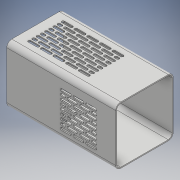
# Autodesk Inventor part: ExtrusionCase
Saved by Autodesk Inventor 2017 (Build 210142000, 142)
## iProperties
Created: 2019-06-19
Part Number: ExtrusionCase
Material: Generic
Document SubType Name: Modeling
Designer: DDeGo
Density: 1 g/cm^3
Appearance: Default
Author: DDeGo
Autodesk Inventor part; units mm, degrees
(part 1 of 2)
ref_plane "YZ Plane" through (0, 0, 0) normal (1, 0, 0) x (0, 1, 0)
ref_plane "XZ Plane" through (0, 0, 0) normal (0, 1, 0) x (-1, 0, 0)
ref_plane "XY Plane" through (0, 0, 0) normal (0, 0, 1) x (1, 0, 0)
sketch "Sketch1" plane through (0, 0, 0) normal (1, 0, 0) x (0, 1, 0)
  line L0 (13, 0) -> (170, 0)
  line L1 (183, -13) -> (183, -170)
  line L2 (170, -183) -> (13, -183)
  line L3 (0, -170) -> (0, -13)
  arc A0 (183, -13) -> (170, 0) centre (170, -13) ccw
  arc A1 (170, -183) -> (183, -170) centre (170, -170) ccw
  arc A2 (0, -170) -> (13, -183) centre (13, -170) ccw
  arc A3 (13, 0) -> (0, -13) centre (13, -13) ccw
  line L4 (186.5, -170) -> (186.5, -13)
  arc A4 (186.5, -13) -> (170, 3.5) centre (170, -13) ccw
  line L5 (170, 3.5) -> (13, 3.5)
  arc A5 (13, 3.5) -> (-3.5, -13) centre (13, -13) ccw
  line L6 (-3.5, -13) -> (-3.5, -170)
  arc A6 (-3.5, -170) -> (13, -186.5) centre (13, -170) ccw
  line L7 (13, -186.5) -> (170, -186.5)
  arc A7 (170, -186.5) -> (186.5, -170) centre (170, -170) ccw
  point P0 (0, 0)
  dimension "d0" = 183
  dimension "d1" = 183
  dimension "d2" = 13
  dimension "d3" = 3.5
  constraints: 16 end point, 16 point on circle, 8 centre point, 8 tangent, 4 parallel, 3 equal radius, 2 perpendicular, 2 point on line, 1 horizontal, 7 other
  measures "d0" distance between parallel lines of L2 L0
  measures "d1" distance between parallel lines of L3 L1
  measures "d2" radius of A0
  measures "d3" distance between parallel lines of L4 L1
extrude "Extrusion1" add sketch "Sketch1" along normal blind 360
sketch "Sketch3" plane through (0, 13, 3.5) normal (0, 0, 1) x (1, 0, 0)
  line L0 (235, 18.5) -> (31, 18.5) construction
  line L1 (31, 18.5) -> (31, 138.5) construction
  line L2 (31, 138.5) -> (235, 138.5) construction
  line L3 (235, 138.5) -> (235, 18.5) construction
  line L4 (0, 157) -> (360, 157) projected
  line L5 (0, 0) -> (360, 0) projected
  line L6 (0, 157) -> (0, 0) projected
  line L7 (230.5556, 134.0556) -> (202.6444, 134.0556) construction
  line L8 (230.5556, 138.5) -> (202.6444, 138.5)
  line L9 (202.6444, 129.6111) -> (230.5556, 129.6111)
  arc A0 (230.5556, 129.6111) -> (230.5556, 138.5) centre (230.5556, 134.0556) ccw
  arc A1 (202.6444, 138.5) -> (202.6444, 129.6111) centre (202.6444, 134.0556) ccw
  line L10 (209.6556, 120.1667) -> (181.7444, 120.1667) construction
  line L11 (209.6556, 124.6111) -> (181.7444, 124.6111)
  line L12 (181.7444, 115.7222) -> (209.6556, 115.7222)
  arc A2 (209.6556, 115.7222) -> (209.6556, 124.6111) centre (209.6556, 120.1667) ccw
  arc A3 (181.7444, 124.6111) -> (181.7444, 115.7222) centre (181.7444, 120.1667) ccw
  arc A4 (202.6444, 110.7222) -> (202.6444, 101.8333) centre (202.6444, 106.2778) ccw
  line L13 (230.5556, 110.7222) -> (202.6444, 110.7222)
  line L14 (202.6444, 101.8333) -> (230.5556, 101.8333)
  arc A5 (230.5556, 101.8333) -> (230.5556, 110.7222) centre (230.5556, 106.2778) ccw
  line L15 (230.5556, 106.2778) -> (202.6444, 106.2778) construction
  arc A6 (202.6444, 82.9444) -> (202.6444, 74.0556) centre (202.6444, 78.5) ccw
  line L16 (230.5556, 82.9444) -> (202.6444, 82.9444)
  line L17 (202.6444, 74.0556) -> (230.5556, 74.0556)
  arc A7 (230.5556, 74.0556) -> (230.5556, 82.9444) centre (230.5556, 78.5) ccw
  line L18 (230.5556, 78.5) -> (202.6444, 78.5) construction
  arc A8 (202.6444, 55.1667) -> (202.6444, 46.2778) centre (202.6444, 50.7222) ccw
  line L19 (230.5556, 55.1667) -> (202.6444, 55.1667)
  line L20 (202.6444, 46.2778) -> (230.5556, 46.2778)
  arc A9 (230.5556, 46.2778) -> (230.5556, 55.1667) centre (230.5556, 50.7222) ccw
  line L21 (230.5556, 50.7222) -> (202.6444, 50.7222) construction
  arc A10 (160.8444, 138.5) -> (160.8444, 129.6111) centre (160.8444, 134.0556) ccw
  line L22 (188.7556, 138.5) -> (160.8444, 138.5)
  line L23 (160.8444, 129.6111) -> (188.7556, 129.6111)
  arc A11 (188.7556, 129.6111) -> (188.7556, 138.5) centre (188.7556, 134.0556) ccw
  line L24 (188.7556, 134.0556) -> (160.8444, 134.0556) construction
  arc A12 (160.8444, 110.7222) -> (160.8444, 101.8333) centre (160.8444, 106.2778) ccw
  line L25 (188.7556, 110.7222) -> (160.8444, 110.7222)
  line L26 (160.8444, 101.8333) -> (188.7556, 101.8333)
  arc A13 (188.7556, 101.8333) -> (188.7556, 110.7222) centre (188.7556, 106.2778) ccw
  line L27 (188.7556, 106.2778) -> (160.8444, 106.2778) construction
  arc A14 (160.8444, 82.9444) -> (160.8444, 74.0556) centre (160.8444, 78.5) ccw
  line L28 (188.7556, 82.9444) -> (160.8444, 82.9444)
  line L29 (160.8444, 74.0556) -> (188.7556, 74.0556)
  arc A15 (188.7556, 74.0556) -> (188.7556, 82.9444) centre (188.7556, 78.5) ccw
  line L30 (188.7556, 78.5) -> (160.8444, 78.5) construction
  arc A16 (160.8444, 55.1667) -> (160.8444, 46.2778) centre (160.8444, 50.7222) ccw
  line L31 (188.7556, 55.1667) -> (160.8444, 55.1667)
  line L32 (160.8444, 46.2778) -> (188.7556, 46.2778)
  arc A17 (188.7556, 46.2778) -> (188.7556, 55.1667) centre (188.7556, 50.7222) ccw
  line L33 (188.7556, 50.7222) -> (160.8444, 50.7222) construction
  arc A18 (119.0444, 138.5) -> (119.0444, 129.6111) centre (119.0444, 134.0556) ccw
  line L34 (146.9556, 138.5) -> (119.0444, 138.5)
  line L35 (119.0444, 129.6111) -> (146.9556, 129.6111)
  arc A19 (146.9556, 129.6111) -> (146.9556, 138.5) centre (146.9556, 134.0556) ccw
  line L36 (146.9556, 134.0556) -> (119.0444, 134.0556) construction
  arc A20 (119.0444, 110.7222) -> (119.0444, 101.8333) centre (119.0444, 106.2778) ccw
  line L37 (146.9556, 110.7222) -> (119.0444, 110.7222)
  line L38 (119.0444, 101.8333) -> (146.9556, 101.8333)
  arc A21 (146.9556, 101.8333) -> (146.9556, 110.7222) centre (146.9556, 106.2778) ccw
  line L39 (146.9556, 106.2778) -> (119.0444, 106.2778) construction
  arc A22 (119.0444, 82.9444) -> (119.0444, 74.0556) centre (119.0444, 78.5) ccw
  line L40 (146.9556, 82.9444) -> (119.0444, 82.9444)
  line L41 (119.0444, 74.0556) -> (146.9556, 74.0556)
  arc A23 (146.9556, 74.0556) -> (146.9556, 82.9444) centre (146.9556, 78.5) ccw
  line L42 (146.9556, 78.5) -> (119.0444, 78.5) construction
  arc A24 (119.0444, 55.1667) -> (119.0444, 46.2778) centre (119.0444, 50.7222) ccw
  line L43 (146.9556, 55.1667) -> (119.0444, 55.1667)
  line L44 (119.0444, 46.2778) -> (146.9556, 46.2778)
  arc A25 (146.9556, 46.2778) -> (146.9556, 55.1667) centre (146.9556, 50.7222) ccw
  line L45 (146.9556, 50.7222) -> (119.0444, 50.7222) construction
  arc A26 (77.2444, 138.5) -> (77.2444, 129.6111) centre (77.2444, 134.0556) ccw
  line L46 (105.1556, 138.5) -> (77.2444, 138.5)
  line L47 (77.2444, 129.6111) -> (105.1556, 129.6111)
  arc A27 (105.1556, 129.6111) -> (105.1556, 138.5) centre (105.1556, 134.0556) ccw
  line L48 (105.1556, 134.0556) -> (77.2444, 134.0556) construction
  arc A28 (77.2444, 110.7222) -> (77.2444, 101.8333) centre (77.2444, 106.2778) ccw
  line L49 (105.1556, 110.7222) -> (77.2444, 110.7222)
  line L50 (77.2444, 101.8333) -> (105.1556, 101.8333)
  arc A29 (105.1556, 101.8333) -> (105.1556, 110.7222) centre (105.1556, 106.2778) ccw
  line L51 (105.1556, 106.2778) -> (77.2444, 106.2778) construction
  arc A30 (77.2444, 82.9444) -> (77.2444, 74.0556) centre (77.2444, 78.5) ccw
  line L52 (105.1556, 82.9444) -> (77.2444, 82.9444)
  line L53 (77.2444, 74.0556) -> (105.1556, 74.0556)
  arc A31 (105.1556, 74.0556) -> (105.1556, 82.9444) centre (105.1556, 78.5) ccw
  line L54 (105.1556, 78.5) -> (77.2444, 78.5) construction
  arc A32 (77.2444, 55.1667) -> (77.2444, 46.2778) centre (77.2444, 50.7222) ccw
  line L55 (105.1556, 55.1667) -> (77.2444, 55.1667)
  line L56 (77.2444, 46.2778) -> (105.1556, 46.2778)
  arc A33 (105.1556, 46.2778) -> (105.1556, 55.1667) centre (105.1556, 50.7222) ccw
  line L57 (105.1556, 50.7222) -> (77.2444, 50.7222) construction
  arc A34 (202.6444, 27.3889) -> (202.6444, 18.5) centre (202.6444, 22.9444) ccw
  line L58 (230.5556, 27.3889) -> (202.6444, 27.3889)
  line L59 (202.6444, 18.5) -> (230.5556, 18.5)
  arc A35 (230.5556, 18.5) -> (230.5556, 27.3889) centre (230.5556, 22.9444) ccw
  line L60 (230.5556, 22.9444) -> (202.6444, 22.9444) construction
  arc A36 (160.8444, 27.3889) -> (160.8444, 18.5) centre (160.8444, 22.9444) ccw
  line L61 (188.7556, 27.3889) -> (160.8444, 27.3889)
  line L62 (160.8444, 18.5) -> (188.7556, 18.5)
  arc A37 (188.7556, 18.5) -> (188.7556, 27.3889) centre (188.7556, 22.9444) ccw
  line L63 (188.7556, 22.9444) -> (160.8444, 22.9444) construction
  arc A38 (119.0444, 27.3889) -> (119.0444, 18.5) centre (119.0444, 22.9444) ccw
  line L64 (146.9556, 27.3889) -> (119.0444, 27.3889)
  line L65 (119.0444, 18.5) -> (146.9556, 18.5)
  arc A39 (146.9556, 18.5) -> (146.9556, 27.3889) centre (146.9556, 22.9444) ccw
  line L66 (146.9556, 22.9444) -> (119.0444, 22.9444) construction
  arc A40 (77.2444, 27.3889) -> (77.2444, 18.5) centre (77.2444, 22.9444) ccw
  line L67 (105.1556, 27.3889) -> (77.2444, 27.3889)
  line L68 (77.2444, 18.5) -> (105.1556, 18.5)
  arc A41 (105.1556, 18.5) -> (105.1556, 27.3889) centre (105.1556, 22.9444) ccw
  line L69 (105.1556, 22.9444) -> (77.2444, 22.9444) construction
  arc A42 (35.4444, 138.5) -> (35.4444, 129.6111) centre (35.4444, 134.0556) ccw
  line L70 (63.3556, 138.5) -> (35.4444, 138.5)
  line L71 (35.4444, 129.6111) -> (63.3556, 129.6111)
  arc A43 (63.3556, 129.6111) -> (63.3556, 138.5) centre (63.3556, 134.0556) ccw
  line L72 (63.3556, 134.0556) -> (35.4444, 134.0556) construction
  arc A44 (35.4444, 110.7222) -> (35.4444, 101.8333) centre (35.4444, 106.2778) ccw
  line L73 (63.3556, 110.7222) -> (35.4444, 110.7222)
  line L74 (35.4444, 101.8333) -> (63.3556, 101.8333)
  arc A45 (63.3556, 101.8333) -> (63.3556, 110.7222) centre (63.3556, 106.2778) ccw
  line L75 (63.3556, 106.2778) -> (35.4444, 106.2778) construction
  arc A46 (35.4444, 82.9444) -> (35.4444, 74.0556) centre (35.4444, 78.5) ccw
  line L76 (63.3556, 82.9444) -> (35.4444, 82.9444)
  line L77 (35.4444, 74.0556) -> (63.3556, 74.0556)
  arc A47 (63.3556, 74.0556) -> (63.3556, 82.9444) centre (63.3556, 78.5) ccw
  line L78 (63.3556, 78.5) -> (35.4444, 78.5) construction
  arc A48 (35.4444, 55.1667) -> (35.4444, 46.2778) centre (35.4444, 50.7222) ccw
  line L79 (63.3556, 55.1667) -> (35.4444, 55.1667)
  line L80 (35.4444, 46.2778) -> (63.3556, 46.2778)
  arc A49 (63.3556, 46.2778) -> (63.3556, 55.1667) centre (63.3556, 50.7222) ccw
  line L81 (63.3556, 50.7222) -> (35.4444, 50.7222) construction
  arc A50 (35.4444, 27.3889) -> (35.4444, 18.5) centre (35.4444, 22.9444) ccw
  line L82 (63.3556, 27.3889) -> (35.4444, 27.3889)
  line L83 (35.4444, 18.5) -> (63.3556, 18.5)
  arc A51 (63.3556, 18.5) -> (63.3556, 27.3889) centre (63.3556, 22.9444) ccw
  line L84 (63.3556, 22.9444) -> (35.4444, 22.9444) construction
  line L85 (216.6, 106.2778) -> (195.7, 120.1667) construction
  line L86 (195.7, 120.1667) -> (174.8, 134.0556) construction
  arc A52 (167.8556, 115.7222) -> (167.8556, 124.6111) centre (167.8556, 120.1667) ccw
  arc A53 (139.9444, 124.6111) -> (139.9444, 115.7222) centre (139.9444, 120.1667) ccw
  line L87 (139.9444, 115.7222) -> (167.8556, 115.7222)
  line L88 (167.8556, 120.1667) -> (139.9444, 120.1667) construction
  line L89 (167.8556, 124.6111) -> (139.9444, 124.6111)
  arc A54 (126.0556, 115.7222) -> (126.0556, 124.6111) centre (126.0556, 120.1667) ccw
  arc A55 (98.1444, 124.6111) -> (98.1444, 115.7222) centre (98.1444, 120.1667) ccw
  line L90 (98.1444, 115.7222) -> (126.0556, 115.7222)
  line L91 (126.0556, 120.1667) -> (98.1444, 120.1667) construction
  line L92 (126.0556, 124.6111) -> (98.1444, 124.6111)
  arc A56 (84.2556, 115.7222) -> (84.2556, 124.6111) centre (84.2556, 120.1667) ccw
  arc A57 (56.3444, 124.6111) -> (56.3444, 115.7222) centre (56.3444, 120.1667) ccw
  line L93 (56.3444, 115.7222) -> (84.2556, 115.7222)
  line L94 (84.2556, 120.1667) -> (56.3444, 120.1667) construction
  line L95 (84.2556, 124.6111) -> (56.3444, 124.6111)
  arc A58 (209.6556, 87.9444) -> (209.6556, 96.8333) centre (209.6556, 92.3889) ccw
  arc A59 (181.7444, 96.8333) -> (181.7444, 87.9444) centre (181.7444, 92.3889) ccw
  line L96 (181.7444, 87.9444) -> (209.6556, 87.9444)
  line L97 (209.6556, 92.3889) -> (181.7444, 92.3889) construction
  line L98 (209.6556, 96.8333) -> (181.7444, 96.8333)
  arc A60 (167.8556, 87.9444) -> (167.8556, 96.8333) centre (167.8556, 92.3889) ccw
  arc A61 (139.9444, 96.8333) -> (139.9444, 87.9444) centre (139.9444, 92.3889) ccw
  line L99 (139.9444, 87.9444) -> (167.8556, 87.9444)
  line L100 (167.8556, 92.3889) -> (139.9444, 92.3889) construction
  line L101 (167.8556, 96.8333) -> (139.9444, 96.8333)
  arc A62 (126.0556, 87.9444) -> (126.0556, 96.8333) centre (126.0556, 92.3889) ccw
  arc A63 (98.1444, 96.8333) -> (98.1444, 87.9444) centre (98.1444, 92.3889) ccw
  line L102 (98.1444, 87.9444) -> (126.0556, 87.9444)
  line L103 (126.0556, 92.3889) -> (98.1444, 92.3889) construction
  line L104 (126.0556, 96.8333) -> (98.1444, 96.8333)
  arc A64 (84.2556, 87.9444) -> (84.2556, 96.8333) centre (84.2556, 92.3889) ccw
  arc A65 (56.3444, 96.8333) -> (56.3444, 87.9444) centre (56.3444, 92.3889) ccw
  line L105 (56.3444, 87.9444) -> (84.2556, 87.9444)
  line L106 (84.2556, 92.3889) -> (56.3444, 92.3889) construction
  line L107 (84.2556, 96.8333) -> (56.3444, 96.8333)
  arc A66 (209.6556, 60.1667) -> (209.6556, 69.0556) centre (209.6556, 64.6111) ccw
  arc A67 (181.7444, 69.0556) -> (181.7444, 60.1667) centre (181.7444, 64.6111) ccw
  line L108 (181.7444, 60.1667) -> (209.6556, 60.1667)
  line L109 (209.6556, 64.6111) -> (181.7444, 64.6111) construction
  line L110 (209.6556, 69.0556) -> (181.7444, 69.0556)
  arc A68 (167.8556, 60.1667) -> (167.8556, 69.0556) centre (167.8556, 64.6111) ccw
  arc A69 (139.9444, 69.0556) -> (139.9444, 60.1667) centre (139.9444, 64.6111) ccw
  line L111 (139.9444, 60.1667) -> (167.8556, 60.1667)
  line L112 (167.8556, 64.6111) -> (139.9444, 64.6111) construction
  line L113 (167.8556, 69.0556) -> (139.9444, 69.0556)
  arc A70 (126.0556, 60.1667) -> (126.0556, 69.0556) centre (126.0556, 64.6111) ccw
  arc A71 (98.1444, 69.0556) -> (98.1444, 60.1667) centre (98.1444, 64.6111) ccw
  line L114 (98.1444, 60.1667) -> (126.0556, 60.1667)
  line L115 (126.0556, 64.6111) -> (98.1444, 64.6111) construction
  line L116 (126.0556, 69.0556) -> (98.1444, 69.0556)
  arc A72 (84.2556, 60.1667) -> (84.2556, 69.0556) centre (84.2556, 64.6111) ccw
  arc A73 (56.3444, 69.0556) -> (56.3444, 60.1667) centre (56.3444, 64.6111) ccw
  line L117 (56.3444, 60.1667) -> (84.2556, 60.1667)
  line L118 (84.2556, 64.6111) -> (56.3444, 64.6111) construction
  line L119 (84.2556, 69.0556) -> (56.3444, 69.0556)
  arc A74 (209.6556, 32.3889) -> (209.6556, 41.2778) centre (209.6556, 36.8333) ccw
  arc A75 (181.7444, 41.2778) -> (181.7444, 32.3889) centre (181.7444, 36.8333) ccw
  line L120 (181.7444, 32.3889) -> (209.6556, 32.3889)
  line L121 (209.6556, 36.8333) -> (181.7444, 36.8333) construction
  line L122 (209.6556, 41.2778) -> (181.7444, 41.2778)
  arc A76 (167.8556, 32.3889) -> (167.8556, 41.2778) centre (167.8556, 36.8333) ccw
  arc A77 (139.9444, 41.2778) -> (139.9444, 32.3889) centre (139.9444, 36.8333) ccw
  line L123 (139.9444, 32.3889) -> (167.8556, 32.3889)
  line L124 (167.8556, 36.8333) -> (139.9444, 36.8333) construction
  line L125 (167.8556, 41.2778) -> (139.9444, 41.2778)
  arc A78 (126.0556, 32.3889) -> (126.0556, 41.2778) centre (126.0556, 36.8333) ccw
  arc A79 (98.1444, 41.2778) -> (98.1444, 32.3889) centre (98.1444, 36.8333) ccw
  line L126 (98.1444, 32.3889) -> (126.0556, 32.3889)
  line L127 (126.0556, 36.8333) -> (98.1444, 36.8333) construction
  line L128 (126.0556, 41.2778) -> (98.1444, 41.2778)
  arc A80 (84.2556, 32.3889) -> (84.2556, 41.2778) centre (84.2556, 36.8333) ccw
  arc A81 (56.3444, 41.2778) -> (56.3444, 32.3889) centre (56.3444, 36.8333) ccw
  line L129 (56.3444, 32.3889) -> (84.2556, 32.3889)
  line L130 (84.2556, 36.8333) -> (56.3444, 36.8333) construction
  line L131 (84.2556, 41.2778) -> (56.3444, 41.2778)
  line L132 (198.2, 134.0556) -> (198.2, 127.2649) construction
  line L133 (193.2, 134.0556) -> (193.2, 126.603) construction
  point P0 (0, -13)
  point P1 (216.6, 134.0556)
  point P2 (235, 110.7222)
  point P3 (235, 82.9444)
  point P4 (216.6, 78.5)
  point P5 (235, 55.1667)
  point P6 (216.6, 50.7222)
  point P7 (193.2, 138.5)
  point P8 (193.2, 110.7222)
  point P9 (174.8, 106.2778)
  point P10 (193.2, 82.9444)
  point P11 (174.8, 78.5)
  point P12 (193.2, 55.1667)
  point P13 (174.8, 50.7222)
  point P14 (151.4, 138.5)
  point P15 (133, 134.0556)
  point P16 (151.4, 110.7222)
  point P17 (133, 106.2778)
  point P18 (151.4, 82.9444)
  point P19 (133, 78.5)
  point P20 (151.4, 55.1667)
  point P21 (133, 50.7222)
  point P22 (109.6, 138.5)
  point P23 (91.2, 134.0556)
  point P24 (109.6, 110.7222)
  point P25 (91.2, 106.2778)
  point P26 (109.6, 82.9444)
  point P27 (91.2, 78.5)
  point P28 (109.6, 55.1667)
  point P29 (91.2, 50.7222)
  point P30 (235, 27.3889)
  point P31 (216.6, 22.9444)
  point P32 (193.2, 27.3889)
  point P33 (174.8, 22.9444)
  point P34 (151.4, 27.3889)
  point P35 (133, 22.9444)
  point P36 (109.6, 27.3889)
  point P37 (91.2, 22.9444)
  point P38 (67.8, 138.5)
  point P39 (49.4, 134.0556)
  point P40 (67.8, 110.7222)
  point P41 (49.4, 106.2778)
  point P42 (67.8, 82.9444)
  point P43 (49.4, 78.5)
  point P44 (67.8, 55.1667)
  point P45 (49.4, 50.7222)
  point P46 (67.8, 27.3889)
  point P47 (49.4, 22.9444)
  point P48 (153.9, 120.1667)
  point P49 (112.1, 120.1667)
  point P50 (70.3, 120.1667)
  point P51 (195.7, 92.3889)
  point P52 (153.9, 92.3889)
  point P53 (112.1, 92.3889)
  point P54 (70.3, 92.3889)
  point P55 (195.7, 64.6111)
  point P56 (153.9, 64.6111)
  point P57 (112.1, 64.6111)
  point P58 (70.3, 64.6111)
  point P59 (195.7, 36.8333)
  point P60 (153.9, 36.8333)
  point P61 (112.1, 36.8333)
  point P62 (70.3, 36.8333)
  dimension "d26" = 18.5
  dimension "d27" = 18.5
  dimension "d28" = 235
  dimension "d29" = 31
  dimension "d37" = 27.7778
  dimension "d40" = 41.8
  dimension "d54" = 41.8
  dimension "d57" = 27.7778
  dimension "d112" = 5
  dimension "d113" = 5
  dimension "d114" = 27.9111
  dimension "d131" = 4.4444
  dimension "d132" = 4.4444
  constraints: 344 end point, 166 point on circle, 82 centre point, 10 tangent, 7 equal length, 5 horizontal, 4 vertical, 2 collinear, 2 midpoint, 1 perpendicular, 492 other
  measures "d26" distance between parallel lines of L2 L4
  measures "d27" distance between parallel lines of L5 L0
  measures "d28" distance between parallel lines of L6 L3
  measures "d29" distance between parallel lines of L6 L1
  measures "d37" distance of L2.end point (235, 110.722)
  measures "d40" distance of L2.end point (193.2, 138.5)
  measures "d54" distance of L10.start L88.start
  measures "d57" distance of L10.start L97.start
  measures "d112" distance between parallel lines of L9 L11
  measures "d113" distance between parallel lines of L133 L132
  measures "d114" distance of L7.start L7.end
  measures "d131" radius of A0
  measures "d132" radius of A2
extrude "Extrusion3" cut sketch "Sketch3" against normal blind 10
sketch "Sketch4" plane through (0, -3.5, -170) normal (0, -1, 0) x (1, 0, 0)
  line L0 (177, 131) -> (297, 131) construction
  line L1 (297, 131) -> (297, 11) construction
  line L2 (297, 11) -> (177, 11) construction
  line L3 (177, 11) -> (177, 131) construction
  line L4 (0, 0) -> (360, 0) projected
  line L5 (0, 157) -> (0, 0) projected
  line L6 (181.4444, 15.4444) -> (209.2222, 15.4444) construction
  line L7 (181.4444, 11) -> (209.2222, 11)
  line L8 (209.2222, 19.8889) -> (181.4444, 19.8889)
  arc A0 (181.4444, 19.8889) -> (181.4444, 11) centre (181.4444, 15.4444) ccw
  arc A1 (209.2222, 11) -> (209.2222, 19.8889) centre (209.2222, 15.4444) ccw
  line L9 (223.1111, 15.4444) -> (250.8889, 15.4444) construction
  line L10 (223.1111, 11) -> (250.8889, 11)
  line L11 (250.8889, 19.8889) -> (223.1111, 19.8889)
  arc A2 (223.1111, 19.8889) -> (223.1111, 11) centre (223.1111, 15.4444) ccw
  arc A3 (250.8889, 11) -> (250.8889, 19.8889) centre (250.8889, 15.4444) ccw
  line L12 (264.7778, 15.4444) -> (292.5556, 15.4444) construction
  line L13 (264.7778, 11) -> (292.5556, 11)
  line L14 (292.5556, 19.8889) -> (264.7778, 19.8889)
  arc A4 (264.7778, 19.8889) -> (264.7778, 11) centre (264.7778, 15.4444) ccw
  arc A5 (292.5556, 11) -> (292.5556, 19.8889) centre (292.5556, 15.4444) ccw
  line L15 (181.4444, 43.2222) -> (209.2222, 43.2222) construction
  line L16 (181.4444, 38.7778) -> (209.2222, 38.7778)
  line L17 (209.2222, 47.6667) -> (181.4444, 47.6667)
  arc A6 (181.4444, 47.6667) -> (181.4444, 38.7778) centre (181.4444, 43.2222) ccw
  arc A7 (209.2222, 38.7778) -> (209.2222, 47.6667) centre (209.2222, 43.2222) ccw
  line L18 (223.1111, 43.2222) -> (250.8889, 43.2222) construction
  line L19 (223.1111, 38.7778) -> (250.8889, 38.7778)
  line L20 (250.8889, 47.6667) -> (223.1111, 47.6667)
  arc A8 (223.1111, 47.6667) -> (223.1111, 38.7778) centre (223.1111, 43.2222) ccw
  arc A9 (250.8889, 38.7778) -> (250.8889, 47.6667) centre (250.8889, 43.2222) ccw
  line L21 (264.7778, 43.2222) -> (292.5556, 43.2222) construction
  line L22 (264.7778, 38.7778) -> (292.5556, 38.7778)
  line L23 (292.5556, 47.6667) -> (264.7778, 47.6667)
  arc A10 (264.7778, 47.6667) -> (264.7778, 38.7778) centre (264.7778, 43.2222) ccw
  arc A11 (292.5556, 38.7778) -> (292.5556, 47.6667) centre (292.5556, 43.2222) ccw
  line L24 (181.4444, 71) -> (209.2222, 71) construction
  line L25 (181.4444, 66.5556) -> (209.2222, 66.5556)
  line L26 (209.2222, 75.4444) -> (181.4444, 75.4444)
  arc A12 (181.4444, 75.4444) -> (181.4444, 66.5556) centre (181.4444, 71) ccw
  arc A13 (209.2222, 66.5556) -> (209.2222, 75.4444) centre (209.2222, 71) ccw
  line L27 (223.1111, 71) -> (250.8889, 71) construction
  line L28 (223.1111, 66.5556) -> (250.8889, 66.5556)
  line L29 (250.8889, 75.4444) -> (223.1111, 75.4444)
  arc A14 (223.1111, 75.4444) -> (223.1111, 66.5556) centre (223.1111, 71) ccw
  arc A15 (250.8889, 66.5556) -> (250.8889, 75.4444) centre (250.8889, 71) ccw
  line L30 (264.7778, 71) -> (292.5556, 71) construction
  line L31 (264.7778, 66.5556) -> (292.5556, 66.5556)
  line L32 (292.5556, 75.4444) -> (264.7778, 75.4444)
  arc A16 (264.7778, 75.4444) -> (264.7778, 66.5556) centre (264.7778, 71) ccw
  arc A17 (292.5556, 66.5556) -> (292.5556, 75.4444) centre (292.5556, 71) ccw
  line L33 (181.4444, 98.7778) -> (209.2222, 98.7778) construction
  line L34 (181.4444, 94.3333) -> (209.2222, 94.3333)
  line L35 (209.2222, 103.2222) -> (181.4444, 103.2222)
  arc A18 (181.4444, 103.2222) -> (181.4444, 94.3333) centre (181.4444, 98.7778) ccw
  arc A19 (209.2222, 94.3333) -> (209.2222, 103.2222) centre (209.2222, 98.7778) ccw
  line L36 (223.1111, 98.7778) -> (250.8889, 98.7778) construction
  line L37 (223.1111, 94.3333) -> (250.8889, 94.3333)
  line L38 (250.8889, 103.2222) -> (223.1111, 103.2222)
  arc A20 (223.1111, 103.2222) -> (223.1111, 94.3333) centre (223.1111, 98.7778) ccw
  arc A21 (250.8889, 94.3333) -> (250.8889, 103.2222) centre (250.8889, 98.7778) ccw
  line L39 (264.7778, 98.7778) -> (292.5556, 98.7778) construction
  line L40 (264.7778, 94.3333) -> (292.5556, 94.3333)
  line L41 (292.5556, 103.2222) -> (264.7778, 103.2222)
  arc A22 (264.7778, 103.2222) -> (264.7778, 94.3333) centre (264.7778, 98.7778) ccw
  arc A23 (292.5556, 94.3333) -> (292.5556, 103.2222) centre (292.5556, 98.7778) ccw
  line L42 (181.4444, 126.5556) -> (209.2222, 126.5556) construction
  line L43 (181.4444, 122.1111) -> (209.2222, 122.1111)
  line L44 (209.2222, 131) -> (181.4444, 131)
  arc A24 (181.4444, 131) -> (181.4444, 122.1111) centre (181.4444, 126.5556) ccw
  arc A25 (209.2222, 122.1111) -> (209.2222, 131) centre (209.2222, 126.5556) ccw
  line L45 (223.1111, 126.5556) -> (250.8889, 126.5556) construction
  line L46 (223.1111, 122.1111) -> (250.8889, 122.1111)
  line L47 (250.8889, 131) -> (223.1111, 131)
  arc A26 (223.1111, 131) -> (223.1111, 122.1111) centre (223.1111, 126.5556) ccw
  arc A27 (250.8889, 122.1111) -> (250.8889, 131) centre (250.8889, 126.5556) ccw
  line L48 (264.7778, 126.5556) -> (292.5556, 126.5556) construction
  line L49 (264.7778, 122.1111) -> (292.5556, 122.1111)
  line L50 (292.5556, 131) -> (264.7778, 131)
  arc A28 (264.7778, 131) -> (264.7778, 122.1111) centre (264.7778, 126.5556) ccw
  arc A29 (292.5556, 122.1111) -> (292.5556, 131) centre (292.5556, 126.5556) ccw
  line L51 (203.6667, 29.3333) -> (228.6667, 29.3333) construction
  line L52 (203.6667, 24.8889) -> (228.6667, 24.8889)
  line L53 (228.6667, 33.7778) -> (203.6667, 33.7778)
  arc A30 (203.6667, 33.7778) -> (203.6667, 24.8889) centre (203.6667, 29.3333) ccw
  arc A31 (228.6667, 24.8889) -> (228.6667, 33.7778) centre (228.6667, 29.3333) ccw
  line L54 (195.3333, 43.2222) -> (216.1667, 29.3333) construction
  line L55 (216.1667, 29.3333) -> (237, 15.4444) construction
  arc A32 (270.3333, 24.8889) -> (270.3333, 33.7778) centre (270.3333, 29.3333) ccw
  line L56 (245.3333, 24.8889) -> (270.3333, 24.8889)
  line L57 (245.3333, 29.3333) -> (270.3333, 29.3333) construction
  line L58 (270.3333, 33.7778) -> (245.3333, 33.7778)
  arc A33 (245.3333, 33.7778) -> (245.3333, 24.8889) centre (245.3333, 29.3333) ccw
  arc A34 (228.6667, 52.6667) -> (228.6667, 61.5556) centre (228.6667, 57.1111) ccw
  line L59 (203.6667, 52.6667) -> (228.6667, 52.6667)
  line L60 (203.6667, 57.1111) -> (228.6667, 57.1111) construction
  line L61 (228.6667, 61.5556) -> (203.6667, 61.5556)
  arc A35 (203.6667, 61.5556) -> (203.6667, 52.6667) centre (203.6667, 57.1111) ccw
  arc A36 (270.3333, 52.6667) -> (270.3333, 61.5556) centre (270.3333, 57.1111) ccw
  line L62 (245.3333, 52.6667) -> (270.3333, 52.6667)
  line L63 (245.3333, 57.1111) -> (270.3333, 57.1111) construction
  line L64 (270.3333, 61.5556) -> (245.3333, 61.5556)
  arc A37 (245.3333, 61.5556) -> (245.3333, 52.6667) centre (245.3333, 57.1111) ccw
  arc A38 (228.6667, 80.4444) -> (228.6667, 89.3333) centre (228.6667, 84.8889) ccw
  line L65 (203.6667, 80.4444) -> (228.6667, 80.4444)
  line L66 (203.6667, 84.8889) -> (228.6667, 84.8889) construction
  line L67 (228.6667, 89.3333) -> (203.6667, 89.3333)
  arc A39 (203.6667, 89.3333) -> (203.6667, 80.4444) centre (203.6667, 84.8889) ccw
  arc A40 (270.3333, 80.4444) -> (270.3333, 89.3333) centre (270.3333, 84.8889) ccw
  line L68 (245.3333, 80.4444) -> (270.3333, 80.4444)
  line L69 (245.3333, 84.8889) -> (270.3333, 84.8889) construction
  line L70 (270.3333, 89.3333) -> (245.3333, 89.3333)
  arc A41 (245.3333, 89.3333) -> (245.3333, 80.4444) centre (245.3333, 84.8889) ccw
  arc A42 (228.6667, 108.2222) -> (228.6667, 117.1111) centre (228.6667, 112.6667) ccw
  line L71 (203.6667, 108.2222) -> (228.6667, 108.2222)
  line L72 (203.6667, 112.6667) -> (228.6667, 112.6667) construction
  line L73 (228.6667, 117.1111) -> (203.6667, 117.1111)
  arc A43 (203.6667, 117.1111) -> (203.6667, 108.2222) centre (203.6667, 112.6667) ccw
  arc A44 (270.3333, 108.2222) -> (270.3333, 117.1111) centre (270.3333, 112.6667) ccw
  line L74 (245.3333, 108.2222) -> (270.3333, 108.2222)
  line L75 (245.3333, 112.6667) -> (270.3333, 112.6667) construction
  line L76 (270.3333, 117.1111) -> (245.3333, 117.1111)
  arc A45 (245.3333, 117.1111) -> (245.3333, 108.2222) centre (245.3333, 112.6667) ccw
  line L77 (213.6667, 15.4444) -> (213.6667, 19.5521) construction
  line L78 (218.6667, 15.4444) -> (218.6667, 18.8098) construction
  point P0 (0, 170)
  point P1 (195.3333, 15.4444)
  point P2 (218.6667, 11)
  point P3 (260.3333, 11)
  point P4 (278.6667, 15.4444)
  point P5 (177, 38.7778)
  point P6 (218.6667, 38.7778)
  point P7 (237, 43.2222)
  point P8 (260.3333, 38.7778)
  point P9 (278.6667, 43.2222)
  point P10 (177, 66.5556)
  point P11 (195.3333, 71)
  point P12 (218.6667, 66.5556)
  point P13 (237, 71)
  point P14 (260.3333, 66.5556)
  point P15 (278.6667, 71)
  point P16 (177, 94.3333)
  point P17 (195.3333, 98.7778)
  point P18 (218.6667, 94.3333)
  point P19 (237, 98.7778)
  point P20 (260.3333, 94.3333)
  point P21 (278.6667, 98.7778)
  point P22 (177, 122.1111)
  point P23 (195.3333, 126.5556)
  point P24 (218.6667, 122.1111)
  point P25 (237, 126.5556)
  point P26 (260.3333, 122.1111)
  point P27 (278.6667, 126.5556)
  point P28 (257.8333, 29.3333)
  point P29 (216.1667, 57.1111)
  point P30 (257.8333, 57.1111)
  point P31 (216.1667, 84.8889)
  point P32 (257.8333, 84.8889)
  point P33 (216.1667, 112.6667)
  point P34 (257.8333, 112.6667)
  dimension "d60" = 120
  dimension "d61" = 120
  dimension "d62" = 11
  dimension "d63" = 177
  dimension "d68" = 41.6667
  dimension "d71" = 27.7778
  dimension "d74" = 25
  dimension "d78" = 41.6667
  dimension "d81" = 27.7778
  dimension "d110" = 5
  dimension "d111" = 27.7778
  dimension "d128" = 5
  dimension "d129" = 4.4444
  dimension "d130" = 4.4444
  constraints: 200 end point, 94 point on circle, 46 centre point, 11 tangent, 5 equal length, 5 horizontal, 4 vertical, 3 collinear, 2 midpoint, 1 perpendicular, 266 other
  measures "d60" distance between parallel lines of L3 L1
  measures "d61" distance between parallel lines of L0 L2
  measures "d62" distance between parallel lines of L4 L2
  measures "d63" distance between parallel lines of L5 L3
  measures "d68" distance of L2.end point (218.667, 11)
  measures "d71" distance of L2.end point (177, 38.778)
  measures "d74" distance of L51.start L51.end
  measures "d78" distance of L52.end L56.end
  measures "d81" distance of L52.end L59.end
  measures "d110" distance between parallel lines of L78 L77
  measures "d111" distance of L6.start L6.end
  measures "d128" distance between parallel lines of L8 L52
  measures "d129" radius of A0
  measures "d130" radius of A30
extrude "Extrusion4" cut sketch "Sketch4" against normal blind 10
sketch "Sketch5" plane through (0, 13, -186.5) normal (0, 0, -1) x (-1, 0, 0)
  line L0 (-12, 10) -> (-142, 10) construction
  line L1 (-142, 10) -> (-142, 147) construction
  line L2 (-142, 147) -> (-12, 147) construction
  line L3 (-12, 147) -> (-12, 10) construction
  line L4 (0, 0) -> (-360, 0) projected
  line L5 (0, 157) -> (-360, 157) projected
  line L6 (0, 0) -> (0, 157) projected
  line L7 (-138.0455, 13.9545) -> (-105.9545, 13.9545) construction
  line L8 (-138.0455, 10) -> (-105.9545, 10)
  line L9 (-105.9545, 17.9091) -> (-138.0455, 17.9091)
  arc A0 (-138.0455, 17.9091) -> (-138.0455, 10) centre (-138.0455, 13.9545) ccw
  arc A1 (-105.9545, 10) -> (-105.9545, 17.9091) centre (-105.9545, 13.9545) ccw
  line L10 (-115.5455, 26.8636) -> (-83.4545, 26.8636) construction
  line L11 (-77.2444, 27.3889) -> (-105.1556, 27.3889) construction
  line L12 (-115.5455, 22.9091) -> (-83.4545, 22.9091)
  line L13 (-83.4545, 30.8182) -> (-115.5455, 30.8182)
  arc A2 (-115.5455, 30.8182) -> (-115.5455, 22.9091) centre (-115.5455, 26.8636) ccw
  arc A3 (-83.4545, 22.9091) -> (-83.4545, 30.8182) centre (-83.4545, 26.8636) ccw
  arc A4 (-60.9545, 10) -> (-60.9545, 17.9091) centre (-60.9545, 13.9545) ccw
  line L14 (-60.9545, 17.9091) -> (-93.0455, 17.9091)
  line L15 (-93.0455, 13.9545) -> (-60.9545, 13.9545) construction
  line L16 (-93.0455, 10) -> (-60.9545, 10)
  arc A5 (-93.0455, 17.9091) -> (-93.0455, 10) centre (-93.0455, 13.9545) ccw
  arc A6 (-105.9545, 35.8182) -> (-105.9545, 43.7273) centre (-105.9545, 39.7727) ccw
  line L17 (-105.9545, 43.7273) -> (-138.0455, 43.7273)
  line L18 (-138.0455, 39.7727) -> (-105.9545, 39.7727) construction
  line L19 (-138.0455, 35.8182) -> (-105.9545, 35.8182)
  arc A7 (-138.0455, 43.7273) -> (-138.0455, 35.8182) centre (-138.0455, 39.7727) ccw
  arc A8 (-60.9545, 35.8182) -> (-60.9545, 43.7273) centre (-60.9545, 39.7727) ccw
  line L20 (-60.9545, 43.7273) -> (-93.0455, 43.7273)
  line L21 (-93.0455, 39.7727) -> (-60.9545, 39.7727) construction
  line L22 (-93.0455, 35.8182) -> (-60.9545, 35.8182)
  arc A9 (-93.0455, 43.7273) -> (-93.0455, 35.8182) centre (-93.0455, 39.7727) ccw
  arc A10 (-15.9545, 10) -> (-15.9545, 17.9091) centre (-15.9545, 13.9545) ccw
  line L23 (-15.9545, 17.9091) -> (-48.0455, 17.9091)
  line L24 (-48.0455, 13.9545) -> (-15.9545, 13.9545) construction
  line L25 (-48.0455, 10) -> (-15.9545, 10)
  arc A11 (-48.0455, 17.9091) -> (-48.0455, 10) centre (-48.0455, 13.9545) ccw
  arc A12 (-15.9545, 35.8182) -> (-15.9545, 43.7273) centre (-15.9545, 39.7727) ccw
  line L26 (-15.9545, 43.7273) -> (-48.0455, 43.7273)
  line L27 (-48.0455, 39.7727) -> (-15.9545, 39.7727) construction
  line L28 (-48.0455, 35.8182) -> (-15.9545, 35.8182)
  arc A13 (-48.0455, 43.7273) -> (-48.0455, 35.8182) centre (-48.0455, 39.7727) ccw
  arc A14 (-105.9545, 61.6364) -> (-105.9545, 69.5455) centre (-105.9545, 65.5909) ccw
  line L29 (-105.9545, 69.5455) -> (-138.0455, 69.5455)
  line L30 (-138.0455, 65.5909) -> (-105.9545, 65.5909) construction
  line L31 (-138.0455, 61.6364) -> (-105.9545, 61.6364)
  arc A15 (-138.0455, 69.5455) -> (-138.0455, 61.6364) centre (-138.0455, 65.5909) ccw
  arc A16 (-60.9545, 61.6364) -> (-60.9545, 69.5455) centre (-60.9545, 65.5909) ccw
  line L32 (-60.9545, 69.5455) -> (-93.0455, 69.5455)
  line L33 (-93.0455, 65.5909) -> (-60.9545, 65.5909) construction
  line L34 (-93.0455, 61.6364) -> (-60.9545, 61.6364)
  arc A17 (-93.0455, 69.5455) -> (-93.0455, 61.6364) centre (-93.0455, 65.5909) ccw
  arc A18 (-15.9545, 61.6364) -> (-15.9545, 69.5455) centre (-15.9545, 65.5909) ccw
  line L35 (-15.9545, 69.5455) -> (-48.0455, 69.5455)
  line L36 (-48.0455, 65.5909) -> (-15.9545, 65.5909) construction
  line L37 (-48.0455, 61.6364) -> (-15.9545, 61.6364)
  arc A19 (-48.0455, 69.5455) -> (-48.0455, 61.6364) centre (-48.0455, 65.5909) ccw
  arc A20 (-105.9545, 87.4545) -> (-105.9545, 95.3636) centre (-105.9545, 91.4091) ccw
  line L38 (-105.9545, 95.3636) -> (-138.0455, 95.3636)
  line L39 (-138.0455, 91.4091) -> (-105.9545, 91.4091) construction
  line L40 (-138.0455, 87.4545) -> (-105.9545, 87.4545)
  arc A21 (-138.0455, 95.3636) -> (-138.0455, 87.4545) centre (-138.0455, 91.4091) ccw
  arc A22 (-60.9545, 87.4545) -> (-60.9545, 95.3636) centre (-60.9545, 91.4091) ccw
  line L41 (-60.9545, 95.3636) -> (-93.0455, 95.3636)
  line L42 (-93.0455, 91.4091) -> (-60.9545, 91.4091) construction
  line L43 (-93.0455, 87.4545) -> (-60.9545, 87.4545)
  arc A23 (-93.0455, 95.3636) -> (-93.0455, 87.4545) centre (-93.0455, 91.4091) ccw
  arc A24 (-15.9545, 87.4545) -> (-15.9545, 95.3636) centre (-15.9545, 91.4091) ccw
  line L44 (-15.9545, 95.3636) -> (-48.0455, 95.3636)
  line L45 (-48.0455, 91.4091) -> (-15.9545, 91.4091) construction
  line L46 (-48.0455, 87.4545) -> (-15.9545, 87.4545)
  arc A25 (-48.0455, 95.3636) -> (-48.0455, 87.4545) centre (-48.0455, 91.4091) ccw
  arc A26 (-105.9545, 113.2727) -> (-105.9545, 121.1818) centre (-105.9545, 117.2273) ccw
  line L47 (-105.9545, 121.1818) -> (-138.0455, 121.1818)
  line L48 (-138.0455, 117.2273) -> (-105.9545, 117.2273) construction
  line L49 (-138.0455, 113.2727) -> (-105.9545, 113.2727)
  arc A27 (-138.0455, 121.1818) -> (-138.0455, 113.2727) centre (-138.0455, 117.2273) ccw
  arc A28 (-60.9545, 113.2727) -> (-60.9545, 121.1818) centre (-60.9545, 117.2273) ccw
  line L50 (-60.9545, 121.1818) -> (-93.0455, 121.1818)
  line L51 (-93.0455, 117.2273) -> (-60.9545, 117.2273) construction
  line L52 (-93.0455, 113.2727) -> (-60.9545, 113.2727)
  arc A29 (-93.0455, 121.1818) -> (-93.0455, 113.2727) centre (-93.0455, 117.2273) ccw
  arc A30 (-15.9545, 113.2727) -> (-15.9545, 121.1818) centre (-15.9545, 117.2273) ccw
  line L53 (-15.9545, 121.1818) -> (-48.0455, 121.1818)
  line L54 (-48.0455, 117.2273) -> (-15.9545, 117.2273) construction
  line L55 (-48.0455, 113.2727) -> (-15.9545, 113.2727)
  arc A31 (-48.0455, 121.1818) -> (-48.0455, 113.2727) centre (-48.0455, 117.2273) ccw
  arc A32 (-105.9545, 139.0909) -> (-105.9545, 147) centre (-105.9545, 143.0455) ccw
  line L56 (-105.9545, 147) -> (-138.0455, 147)
  line L57 (-138.0455, 143.0455) -> (-105.9545, 143.0455) construction
  line L58 (-138.0455, 139.0909) -> (-105.9545, 139.0909)
  arc A33 (-138.0455, 147) -> (-138.0455, 139.0909) centre (-138.0455, 143.0455) ccw
  arc A34 (-60.9545, 139.0909) -> (-60.9545, 147) centre (-60.9545, 143.0455) ccw
  line L59 (-60.9545, 147) -> (-93.0455, 147)
  line L60 (-93.0455, 143.0455) -> (-60.9545, 143.0455) construction
  line L61 (-93.0455, 139.0909) -> (-60.9545, 139.0909)
  arc A35 (-93.0455, 147) -> (-93.0455, 139.0909) centre (-93.0455, 143.0455) ccw
  arc A36 (-15.9545, 139.0909) -> (-15.9545, 147) centre (-15.9545, 143.0455) ccw
  line L62 (-15.9545, 147) -> (-48.0455, 147)
  line L63 (-48.0455, 143.0455) -> (-15.9545, 143.0455) construction
  line L64 (-48.0455, 139.0909) -> (-15.9545, 139.0909)
  arc A37 (-48.0455, 147) -> (-48.0455, 139.0909) centre (-48.0455, 143.0455) ccw
  line L65 (-122, 39.7727) -> (-99.5, 26.8636) construction
  line L66 (-99.5, 26.8636) -> (-77, 13.9545) construction
  line L67 (-70.5455, 26.8636) -> (-38.4545, 26.8636) construction
  line L68 (-70.5455, 22.9091) -> (-38.4545, 22.9091)
  line L69 (-38.4545, 30.8182) -> (-70.5455, 30.8182)
  arc A38 (-70.5455, 30.8182) -> (-70.5455, 22.9091) centre (-70.5455, 26.8636) ccw
  arc A39 (-38.4545, 22.9091) -> (-38.4545, 30.8182) centre (-38.4545, 26.8636) ccw
  line L70 (-115.5455, 52.6818) -> (-83.4545, 52.6818) construction
  line L71 (-115.5455, 48.7273) -> (-83.4545, 48.7273)
  line L72 (-83.4545, 56.6364) -> (-115.5455, 56.6364)
  arc A40 (-115.5455, 56.6364) -> (-115.5455, 48.7273) centre (-115.5455, 52.6818) ccw
  arc A41 (-83.4545, 48.7273) -> (-83.4545, 56.6364) centre (-83.4545, 52.6818) ccw
  line L73 (-70.5455, 52.6818) -> (-38.4545, 52.6818) construction
  line L74 (-70.5455, 48.7273) -> (-38.4545, 48.7273)
  line L75 (-38.4545, 56.6364) -> (-70.5455, 56.6364)
  arc A42 (-70.5455, 56.6364) -> (-70.5455, 48.7273) centre (-70.5455, 52.6818) ccw
  arc A43 (-38.4545, 48.7273) -> (-38.4545, 56.6364) centre (-38.4545, 52.6818) ccw
  line L76 (-115.5455, 78.5) -> (-83.4545, 78.5) construction
  line L77 (-115.5455, 74.5455) -> (-83.4545, 74.5455)
  line L78 (-83.4545, 82.4545) -> (-115.5455, 82.4545)
  arc A44 (-115.5455, 82.4545) -> (-115.5455, 74.5455) centre (-115.5455, 78.5) ccw
  arc A45 (-83.4545, 74.5455) -> (-83.4545, 82.4545) centre (-83.4545, 78.5) ccw
  line L79 (-70.5455, 78.5) -> (-38.4545, 78.5) construction
  line L80 (-70.5455, 74.5455) -> (-38.4545, 74.5455)
  line L81 (-38.4545, 82.4545) -> (-70.5455, 82.4545)
  arc A46 (-70.5455, 82.4545) -> (-70.5455, 74.5455) centre (-70.5455, 78.5) ccw
  arc A47 (-38.4545, 74.5455) -> (-38.4545, 82.4545) centre (-38.4545, 78.5) ccw
  line L82 (-115.5455, 104.3182) -> (-83.4545, 104.3182) construction
  line L83 (-115.5455, 100.3636) -> (-83.4545, 100.3636)
  line L84 (-83.4545, 108.2727) -> (-115.5455, 108.2727)
  arc A48 (-115.5455, 108.2727) -> (-115.5455, 100.3636) centre (-115.5455, 104.3182) ccw
  arc A49 (-83.4545, 100.3636) -> (-83.4545, 108.2727) centre (-83.4545, 104.3182) ccw
  line L85 (-70.5455, 104.3182) -> (-38.4545, 104.3182) construction
  line L86 (-70.5455, 100.3636) -> (-38.4545, 100.3636)
  line L87 (-38.4545, 108.2727) -> (-70.5455, 108.2727)
  arc A50 (-70.5455, 108.2727) -> (-70.5455, 100.3636) centre (-70.5455, 104.3182) ccw
  arc A51 (-38.4545, 100.3636) -> (-38.4545, 108.2727) centre (-38.4545, 104.3182) ccw
  line L88 (-115.5455, 130.1364) -> (-83.4545, 130.1364) construction
  line L89 (-115.5455, 126.1818) -> (-83.4545, 126.1818)
  line L90 (-83.4545, 134.0909) -> (-115.5455, 134.0909)
  arc A52 (-115.5455, 134.0909) -> (-115.5455, 126.1818) centre (-115.5455, 130.1364) ccw
  arc A53 (-83.4545, 126.1818) -> (-83.4545, 134.0909) centre (-83.4545, 130.1364) ccw
  line L91 (-70.5455, 130.1364) -> (-38.4545, 130.1364) construction
  line L92 (-70.5455, 126.1818) -> (-38.4545, 126.1818)
  line L93 (-38.4545, 134.0909) -> (-70.5455, 134.0909)
  arc A54 (-70.5455, 134.0909) -> (-70.5455, 126.1818) centre (-70.5455, 130.1364) ccw
  arc A55 (-38.4545, 126.1818) -> (-38.4545, 134.0909) centre (-38.4545, 130.1364) ccw
  line L94 (-102, 13.9545) -> (-102, 22.25) construction
  line L95 (-97, 13.9545) -> (-97, 20.9047) construction
  point P0 (0, -13)
  point P1 (-122, 13.9545)
  point P2 (-97, 10)
  point P3 (-142, 35.8182)
  point P4 (-77, 39.7727)
  point P5 (-97, 35.8182)
  point P6 (-32, 13.9545)
  point P7 (-52, 10)
  point P8 (-32, 39.7727)
  point P9 (-52, 35.8182)
  point P10 (-122, 65.5909)
  point P11 (-142, 61.6364)
  point P12 (-77, 65.5909)
  point P13 (-97, 61.6364)
  point P14 (-32, 65.5909)
  point P15 (-52, 61.6364)
  point P16 (-122, 91.4091)
  point P17 (-142, 87.4545)
  point P18 (-77, 91.4091)
  point P19 (-97, 87.4545)
  point P20 (-32, 91.4091)
  point P21 (-52, 87.4545)
  point P22 (-122, 117.2273)
  point P23 (-142, 113.2727)
  point P24 (-77, 117.2273)
  point P25 (-97, 113.2727)
  point P26 (-32, 117.2273)
  point P27 (-52, 113.2727)
  point P28 (-122, 143.0455)
  point P29 (-142, 139.0909)
  point P30 (-77, 143.0455)
  point P31 (-97, 139.0909)
  point P32 (-32, 143.0455)
  point P33 (-52, 139.0909)
  point P34 (-60.1556, 27.3889)
  point P35 (-54.5, 26.8636)
  point P36 (-105.1556, 53.2071)
  point P37 (-99.5, 52.6818)
  point P38 (-60.1556, 53.2071)
  point P39 (-54.5, 52.6818)
  point P40 (-105.1556, 79.0253)
  point P41 (-99.5, 78.5)
  point P42 (-60.1556, 79.0253)
  point P43 (-54.5, 78.5)
  point P44 (-105.1556, 104.8434)
  point P45 (-99.5, 104.3182)
  point P46 (-60.1556, 104.8434)
  point P47 (-54.5, 104.3182)
  point P48 (-105.1556, 130.6616)
  point P49 (-99.5, 130.1364)
  point P50 (-60.1556, 130.6616)
  point P51 (-54.5, 130.1364)
  dimension "d84" = 10
  dimension "d85" = 10
  dimension "d86" = 12
  dimension "d87" = 130
  dimension "d95" = 45
  dimension "d98" = 25.8182
  dimension "d103" = 45
  dimension "d106" = 25.8182
  dimension "d145" = 5
  dimension "d146" = 3.9545
  dimension "d148" = 5
  constraints: 240 end point, 114 point on circle, 56 centre point, 10 tangent, 5 parallel, 4 horizontal, 4 vertical, 3 collinear, 2 equal length, 2 midpoint, 1 equal radius, 1 perpendicular, 338 other
  measures "d84" distance between parallel lines of L4 L0
  measures "d85" distance between parallel lines of L5 L2
  measures "d86" distance between parallel lines of L6 L3
  measures "d87" distance between parallel lines of L3 L1
  measures "d95" distance of L7.end L15.end
  measures "d98" distance of L7.end L18.end
  measures "d103" distance of L12.start L68.start
  measures "d106" distance of L12.start L71.start
  measures "d145" distance between parallel lines of L94 L95
  measures "d146" radius of A0
  measures "d148" distance between parallel lines of L12 L9
extrude "Extrusion5" cut sketch "Sketch5" against normal blind 10
sketch "Sketch7" plane through (0, -3.5, -170) normal (0, -1, 0) x (1, 0, 0)
  line L0 (181.4444, 29.3333) -> (189.7778, 29.3333) construction
  line L1 (181.4444, 24.8889) -> (189.7778, 24.8889)
  line L2 (189.7778, 33.7778) -> (181.4444, 33.7778)
  arc A0 (181.4444, 33.7778) -> (181.4444, 24.8889) centre (181.4444, 29.3333) ccw
  arc A1 (189.7778, 24.8889) -> (189.7778, 33.7778) centre (189.7778, 29.3333) ccw
  arc A2 (181.4444, 47.6667) -> (181.4444, 38.7778) centre (181.4444, 43.2222) ccw projected
  line L3 (181.4444, 29.3333) -> (181.4444, 43.2222) construction
  arc A3 (203.6667, 33.7778) -> (203.6667, 24.8889) centre (203.6667, 29.3333) ccw projected
  line L4 (189.7778, 29.3333) -> (203.6667, 29.3333) construction
  line L5 (209.2222, 38.7778) -> (181.4444, 38.7778) projected
  line L6 (203.6667, 33.7778) -> (228.6667, 33.7778) projected
  line L7 (194.2222, 29.3333) -> (194.2222, 34.6238) construction
  line L8 (199.2222, 29.3333) -> (199.2222, 34.6238) construction
  line L9 (360, 157) -> (360, 0) projected
  arc A4 (292.5556, 24.8889) -> (292.5556, 33.7778) centre (292.5556, 29.3333) ccw
  line L10 (284.2222, 29.3333) -> (292.5556, 29.3333) construction
  line L11 (284.2222, 24.8889) -> (292.5556, 24.8889)
  line L12 (292.5556, 33.7778) -> (284.2222, 33.7778)
  arc A5 (284.2222, 33.7778) -> (284.2222, 24.8889) centre (284.2222, 29.3333) ccw
  arc A6 (189.7778, 52.6667) -> (189.7778, 61.5556) centre (189.7778, 57.1111) ccw
  line L13 (181.4444, 57.1111) -> (189.7778, 57.1111) construction
  line L14 (181.4444, 52.6667) -> (189.7778, 52.6667)
  line L15 (189.7778, 61.5556) -> (181.4444, 61.5556)
  arc A7 (181.4444, 61.5556) -> (181.4444, 52.6667) centre (181.4444, 57.1111) ccw
  arc A8 (292.5556, 52.6667) -> (292.5556, 61.5556) centre (292.5556, 57.1111) ccw
  line L16 (284.2222, 57.1111) -> (292.5556, 57.1111) construction
  line L17 (284.2222, 52.6667) -> (292.5556, 52.6667)
  line L18 (292.5556, 61.5556) -> (284.2222, 61.5556)
  arc A9 (284.2222, 61.5556) -> (284.2222, 52.6667) centre (284.2222, 57.1111) ccw
  arc A10 (189.7778, 80.4444) -> (189.7778, 89.3333) centre (189.7778, 84.8889) ccw
  line L19 (181.4444, 84.8889) -> (189.7778, 84.8889) construction
  line L20 (181.4444, 80.4444) -> (189.7778, 80.4444)
  line L21 (189.7778, 89.3333) -> (181.4444, 89.3333)
  arc A11 (181.4444, 89.3333) -> (181.4444, 80.4444) centre (181.4444, 84.8889) ccw
  arc A12 (292.5556, 80.4444) -> (292.5556, 89.3333) centre (292.5556, 84.8889) ccw
  line L22 (284.2222, 84.8889) -> (292.5556, 84.8889) construction
  line L23 (284.2222, 80.4444) -> (292.5556, 80.4444)
  line L24 (292.5556, 89.3333) -> (284.2222, 89.3333)
  arc A13 (284.2222, 89.3333) -> (284.2222, 80.4444) centre (284.2222, 84.8889) ccw
  arc A14 (189.7778, 108.2222) -> (189.7778, 117.1111) centre (189.7778, 112.6667) ccw
  line L25 (181.4444, 112.6667) -> (189.7778, 112.6667) construction
  line L26 (181.4444, 108.2222) -> (189.7778, 108.2222)
  line L27 (189.7778, 117.1111) -> (181.4444, 117.1111)
  arc A15 (181.4444, 117.1111) -> (181.4444, 108.2222) centre (181.4444, 112.6667) ccw
  arc A16 (292.5556, 108.2222) -> (292.5556, 117.1111) centre (292.5556, 112.6667) ccw
  line L28 (284.2222, 112.6667) -> (292.5556, 112.6667) construction
  line L29 (284.2222, 108.2222) -> (292.5556, 108.2222)
  line L30 (292.5556, 117.1111) -> (284.2222, 117.1111)
  arc A17 (284.2222, 117.1111) -> (284.2222, 108.2222) centre (284.2222, 112.6667) ccw
  arc A18 (292.5556, 38.7778) -> (292.5556, 47.6667) centre (292.5556, 43.2222) ccw projected
  line L31 (292.5556, 43.2222) -> (292.5556, 29.3333) construction
  line L32 (181.4444, 47.6667) -> (209.2222, 47.6667) projected
  point P0 (0, 170)
  point P1 (185.6111, 29.3333)
  point P2 (297, 29.3333)
  point P3 (288.3889, 29.3333)
  point P4 (194.2222, 57.1111)
  point P5 (185.6111, 57.1111)
  point P6 (297, 57.1111)
  point P7 (288.3889, 57.1111)
  point P8 (194.2222, 84.8889)
  point P9 (185.6111, 84.8889)
  point P10 (297, 84.8889)
  point P11 (288.3889, 84.8889)
  point P12 (194.2222, 112.6667)
  point P13 (185.6111, 112.6667)
  point P14 (297, 112.6667)
  point P15 (288.3889, 112.6667)
  dimension "d115" = 5
  dimension "d116" = 5
  dimension "d119" = 102.7778
  dimension "d122" = 27.7778
  dimension "d125" = 5
  constraints: 74 end point, 34 point on circle, 16 centre point, 5 tangent, 4 vertical, 3 horizontal, 2 point on line, 1 equal radius, 1 midpoint, 1 parallel, 1 perpendicular, 91 other
  measures "d115" distance between parallel lines of L5 L6
  measures "d116" distance between parallel lines of L7 L8
  measures "d119" distance of L1.start L11.start
  measures "d122" distance of L1.start L14.start
  measures "d125" distance between parallel lines of L14 L32
extrude "Extrusion7" cut sketch "Sketch7" against normal blind 10